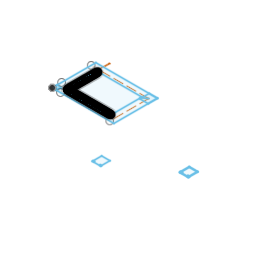
2023_01_21_LaserA4Measure (Autodesk Fusion 360 design; units mm, degrees)
Autodesk Fusion 360 part; units mm, degrees
sketch "Esquisse1" plane through (0, 0, 0) normal (0, 0, 1) x (1, 0, 0)
  line L0 (0, 0) -> (40, 0)
  line L1 (40, 0) -> (40, 45)
  line L2 (40, 45) -> (0, 45)
  line L3 (0, 45) -> (0, 0)
  line L4 (20, 43) -> (20, 40.2)
  line L5 (20, 43) -> (0, 43)
  line L6 (0, 43) -> (0, 45)
  line L7 (0, 45) -> (20, 45)
  line L8 (20, 45) -> (20, 43)
  line L9 (20, 43) -> (40, 43)
  line L10 (40, 43) -> (40, 45)
  line L11 (40, 45) -> (20, 45)
  line L12 (20, 45) -> (20, 43)
  line L13 (20, 43) -> (40, 43)
  line L14 (40, 43) -> (40, 40.2)
  line L15 (40, 40.2) -> (20, 40.2)
  line L16 (20, 40.2) -> (20, 43)
  line L17 (20, 43) -> (0, 43)
  line L18 (0, 43) -> (0, 40.2)
  line L19 (20, 40.2) -> (20, 43)
  line L20 (-0.3, 45.3) -> (-0.3, -0.3)
  line L21 (-0.3, -0.3) -> (40.3, -0.3)
  line L22 (40.3, -0.3) -> (40.3, 45.3)
  line L23 (40.3, 45.3) -> (20, 45.3)
  line L24 (-0.3, 45.3) -> (20, 45.3)
  line L25 (20, 41.6) -> (5.56, 41.6)
  line L26 (20, 41.6) -> (34.44, 41.6)
  line L27 (34.44, 40.2) -> (34.44, 43)
  line L28 (-4.5858, 40) -> (-4.5858, 43)
  line L29 (5.56, 40.2) -> (5.56, 43)
  line L30 (20, 40.2) -> (-0.0001, 40.2)
  dimension "d1" = 40
  dimension "d2" = 45
  dimension "d7" = 2.8
  dimension "d8" = 2
  dimension "d9" = -0.3
  dimension "d10" = 14.44
  dimension "d11" = 14.44
  dimension "d12" = 3
  constraint horizontal L0
  constraint vertical L1
  constraint horizontal L2
  constraint vertical L3
  constraint coincident L0.start L3.end
  constraint vertical L4
  constraint horizontal L5
  constraint vertical L6
  constraint horizontal L7
  constraint vertical L8
  constraint horizontal L9
  constraint vertical L10
  constraint horizontal L11
  constraint vertical L12
  constraint horizontal L13
  constraint vertical L14
  constraint horizontal L15
  constraint vertical L16
  constraint coincident L1 L14.end
  constraint horizontal L17
  constraint vertical L18
  constraint vertical L19
  constraint midpoint L4 L25.start
  constraint perpendicular L16 L25
  constraint perpendicular L19 L26
  constraint coincident L15 L27.start
  constraint perpendicular L15 L27
  constraint coincident L5 L28.end
  constraint perpendicular L5 L28
  constraint coincident L5 L29.end
  constraint perpendicular L5 L29
  constraint horizontal L30
  constraint coincident L30 L29.start
  constraint coincident L30 L18.end
  measures "d1" distance of L0.start L0.end
  measures "d2" distance of L0.start L2.end
  measures "d7" distance of L4.start L4.end
  measures "d8" distance of L4.start L7.end
  measures "d10" distance of L25.start L25.end
  measures "d11" distance of L25.start L26.end
  measures "d12" distance of L28.start L28.end
extrude "Extrusion1" add sketch "Esquisse1" along normal blind 2 contours L0 L1 L3 L15 L30 | L2 L3 L5 L6 L7 L8 L12 L17 | L4 L16 L19 L25 L29 L30 | L1 L2 L8 L9 L10 L11 L12 L13 | L4 L15 L16 L19 L26 L27 | L4 L5 L16 L17 L19 L25 L29 | L4 L9 L13 L16 L19 L26 L27 makes body 1
sketch "Esquisse2" plane through (0, 0, 2) normal (0, 0, 1) x (-1, 0, 0)
  line L0 (0, -40.2) -> (0, 0)
  line L1 (0, 0) -> (-40, 0)
  line L2 (-40, 0) -> (-40, -40.2)
  line L3 (-40, -40.2) -> (-34.44, -40.2)
  line L4 (-34.44, -40.2) -> (-34.44, -43)
  line L5 (-34.44, -43) -> (-40, -43)
  line L6 (-40, -43) -> (-40, -45)
  line L7 (-40, -45) -> (0, -45)
  line L8 (0, -45) -> (0, -43)
  line L9 (0, -43) -> (-5.56, -43)
  line L10 (-5.56, -43) -> (-5.56, -40.2)
  line L11 (-5.56, -40.2) -> (0, -40.2)
  line L12 (-34.74, -40.5) -> (-34.74, -42.7)
  line L13 (-34.74, -42.7) -> (-40.3, -42.7)
  line L14 (-40.3, -42.7) -> (-40.3, -45.3)
  line L15 (-40.3, -45.3) -> (0.3, -45.3)
  line L16 (0.3, -45.3) -> (0.3, -42.7)
  line L17 (0.3, -42.7) -> (-5.26, -42.7)
  line L18 (-5.26, -42.7) -> (-5.26, -40.5)
  line L19 (-5.26, -40.5) -> (0.3, -40.5)
  line L20 (0.3, -40.5) -> (0.3, 0.3)
  line L21 (0.3, 0.3) -> (-40.3, 0.3)
  line L22 (-40.3, 0.3) -> (-40.3, -40.5)
  line L23 (-40.3, -40.5) -> (-34.74, -40.5)
  line L24 (-44, -39) -> (-44, -44.2)
  line L25 (-44, -44.2) -> (-44, -49)
  line L26 (-44, -49) -> (4, -49)
  line L27 (4, -49) -> (4, -44.2)
  line L28 (4, -44.2) -> (4, -39)
  line L29 (4, -39) -> (4, 4)
  line L30 (4, 4) -> (-44, 4)
  line L31 (-44, 4) -> (-44, -39)
  dimension "d15" = 0.3
  dimension "d16" = 4
extrude "Extrusion2" add sketch "Esquisse2" against normal blind 2 separate body contours L24 L25 L26 L27 L28 L29 L30 L31 makes body 2
sketch "Esquisse3" plane through (0, 0, 0) normal (0, 0, 1) x (1, 0, 0)
  line L0 (0, 0) -> (410, 0)
  line L1 (410, 0) -> (410, 400)
  line L2 (410, 400) -> (0, 400)
  line L3 (0, 400) -> (0, 0)
  line L4 (10, 10) -> (400, 10)
  line L5 (400, 10) -> (400, 390)
  line L6 (400, 390) -> (10, 390)
  line L7 (10, 390) -> (10, 10)
  dimension "d19" = 410
  dimension "d20" = 400
  dimension "d21" = -10
  constraint horizontal L0
  constraint vertical L1
  constraint horizontal L2
  constraint vertical L3
  constraint coincident L0.start L3.end
  measures "d19" distance of L0.start L0.end
  measures "d20" distance of L0.start L2.end
move_body "Déplacer1" bodies 1 2 to x (1, 0, 0) y (0, 1, 0) z (0, 0, 1) at (20, 20, 0)
sketch "Esquisse4" plane through (0, 0, 2) normal (0, 0, 1) x (-1, 0, 0)
  line L0 (-20, -60.2) -> (-20, -20)
  line L1 (-20, -20) -> (-60, -20)
  line L2 (-60, -20) -> (-60, -60.2)
  line L3 (-60, -60.2) -> (-54.44, -60.2)
  line L4 (-54.44, -60.2) -> (-54.44, -63)
  line L5 (-54.44, -63) -> (-60, -63)
  line L6 (-60, -63) -> (-60, -65)
  line L7 (-60, -65) -> (-20, -65)
  line L8 (-20, -65) -> (-20, -63)
  line L9 (-20, -63) -> (-25.56, -63)
  line L10 (-25.56, -63) -> (-25.56, -60.2)
  line L11 (-25.56, -60.2) -> (-20, -60.2)
copy_body "Copier/Coller des corps1" bodies 2 1 makes body 3 makes body 4
move_body "Déplacer2" bodies 3 4 to x (1, 0, 0) y (0, 1, 0) z (0, 0, 1) at (300, 300, 0)
sketch "Esquisse5" plane through (0, 0, 0) normal (0, 0, 1) x (1, 0, 0)
  line L0 (-350, 0) -> (-53, 0)
  line L1 (-53, 0) -> (-53, 210)
  line L2 (-53, 210) -> (-350, 210)
  line L3 (-350, 210) -> (-350, 0)
  line L4 (-345, 5) -> (-58, 5)
  line L5 (-58, 5) -> (-58, 205)
  line L6 (-58, 205) -> (-345, 205)
  line L7 (-345, 205) -> (-345, 5)
  line L8 (-305.6385, 29.0688) -> (-95.6385, 29.0688)
  line L9 (-95.6385, 29.0688) -> (-95.6385, 177.5688)
  line L10 (-95.6385, 177.5688) -> (-305.6385, 177.5688)
  line L11 (-305.6385, 177.5688) -> (-305.6385, 29.0688)
  dimension "d28" = 297
  dimension "d29" = 210
  dimension "d30" = -5
  dimension "d31" = 210
  dimension "d32" = 148.5
  constraint horizontal L0
  constraint vertical L1
  constraint horizontal L2
  constraint vertical L3
  constraint horizontal L8
  constraint vertical L9
  constraint horizontal L10
  constraint vertical L11
  measures "d28" distance of L0.start L0.end
  measures "d29" distance of L0.start L2.end
  measures "d31" distance of L8.start L8.end
  measures "d32" distance of L8.start L10.end
copy_body "Copier/Coller des corps2" bodies 1 makes body 5
move_body "Déplacer3" bodies 5 to x (1, 0, 0) y (0, 1, 0) z (0, 0, 1) at (-370, -20, 0)
copy_body "Copier/Coller des corps3" bodies 5 makes body 6
move_body "Déplacer4" bodies 6 to x (1, 0, 0) y (0, 1, 0) z (0, 0, 1) at (257, 165, 0)
sketch "Esquisse7" plane through (0, 0, 2) normal (0, 0, 1) x (-1, 0, 0)
  line L0 (350, -40.2) -> (350, 0)
  line L1 (350, 0) -> (310, 0)
  line L2 (310, 0) -> (310, -40.2)
  line L3 (310, -40.2) -> (315.56, -40.2)
  line L4 (315.56, -40.2) -> (315.56, -43)
  line L5 (315.56, -43) -> (310, -43)
  line L6 (310, -43) -> (310, -45)
  line L7 (310, -45) -> (350, -45)
  line L8 (350, -45) -> (350, -43)
  line L9 (350, -43) -> (344.44, -43)
  line L10 (344.44, -43) -> (344.44, -40.2)
  line L11 (344.44, -40.2) -> (350, -40.2)
  line L12 (350, -43) -> (344.44, -43)
  line L13 (344.44, -43) -> (344.44, -40.2)
  line L14 (344.44, -40.2) -> (350, -40.2)
  line L15 (350, -40.2) -> (350, 0)
  line L16 (350, 0) -> (310, 0)
  line L17 (310, 0) -> (310, -40.2)
  line L18 (310, -40.2) -> (315.56, -40.2)
  line L19 (315.56, -40.2) -> (315.56, -43)
  line L20 (315.56, -43) -> (310, -43)
  line L21 (310, -43) -> (310, -45)
  line L22 (310, -45) -> (350, -45)
  line L23 (350, -45) -> (350, -43)
sketch "Esquisse8" plane through (0, 0, 2) normal (0, 0, 1) x (-1, 0, 0)
  line L0 (93, -205.2) -> (93, -165)
  line L1 (93, -165) -> (53, -165)
  line L2 (53, -165) -> (53, -205.2)
  line L3 (53, -205.2) -> (58.56, -205.2)
  line L4 (58.56, -205.2) -> (58.56, -208)
  line L5 (58.56, -208) -> (53, -208)
  line L6 (53, -208) -> (53, -210)
  line L7 (53, -210) -> (93, -210)
  line L8 (93, -210) -> (93, -208)
  line L9 (93, -208) -> (87.44, -208)
  line L10 (87.44, -208) -> (87.44, -205.2)
  line L11 (87.44, -205.2) -> (93, -205.2)
  line L12 (53, -205.2) -> (58.56, -205.2)
  line L13 (58.56, -205.2) -> (58.56, -208)
  line L14 (58.56, -208) -> (53, -208)
  line L15 (53, -208) -> (53, -210)
  line L16 (53, -210) -> (93, -210)
  line L17 (93, -210) -> (93, -208)
  line L18 (93, -208) -> (87.44, -208)
  line L19 (87.44, -208) -> (87.44, -205.2)
  line L20 (87.44, -205.2) -> (93, -205.2)
  line L21 (93, -205.2) -> (93, -165)
  line L22 (93, -165) -> (53, -165)
  line L23 (53, -165) -> (53, -205.2)
sketch "Esquisse6" plane through (0, 0, 0) normal (0, 0, 1) x (1, 0, 0)
  line L0 (-305.6385, 29.0688) -> (-305.6385, 20)
  line L1 (-295.6385, 29.0688) -> (-295.6385, 20)
  line L2 (-285.6385, 29.0688) -> (-285.6385, 20)
  line L3 (-275.6385, 29.0688) -> (-275.6385, 20)
  line L4 (-265.6385, 29.0688) -> (-265.6385, 20)
  line L5 (-255.6385, 29.0688) -> (-255.6385, 20)
  line L6 (-245.6385, 29.0688) -> (-245.6385, 20)
  line L7 (-235.6385, 29.0688) -> (-235.6385, 20)
  line L8 (-225.6385, 29.0688) -> (-225.6385, 20)
  line L9 (-215.6385, 29.0688) -> (-215.6385, 20)
  line L10 (-205.6385, 29.0688) -> (-205.6385, 20)
  line L11 (-195.6385, 29.0688) -> (-195.6385, 20)
  line L12 (-185.6385, 29.0688) -> (-185.6385, 20)
  line L13 (-175.6385, 29.0688) -> (-175.6385, 20)
  line L14 (-165.6385, 29.0688) -> (-165.6385, 20)
  line L15 (-155.6385, 29.0688) -> (-155.6385, 20)
  line L16 (-145.6385, 29.0688) -> (-145.6385, 20)
  line L17 (-135.6385, 29.0688) -> (-135.6385, 20)
  line L18 (-125.6385, 29.0688) -> (-125.6385, 20)
  line L19 (-115.6385, 29.0688) -> (-115.6385, 20)
  line L20 (-105.6385, 29.0688) -> (-105.6385, 20)
  line L21 (-95.6385, 29.0688) -> (-95.6385, 20)
  line L22 (-305.6385, 29.0688) -> (-305.6385, 27)
  line L23 (-304.6385, 29.0688) -> (-304.6385, 27)
  line L24 (-303.6385, 29.0688) -> (-303.6385, 27)
  line L25 (-302.6385, 29.0688) -> (-302.6385, 27)
  line L26 (-301.6385, 29.0688) -> (-301.6385, 27)
  line L27 (-300.6385, 29.0688) -> (-300.6385, 27)
  line L28 (-299.6385, 29.0688) -> (-299.6385, 27)
  line L29 (-298.6385, 29.0688) -> (-298.6385, 27)
  line L30 (-297.6385, 29.0688) -> (-297.6385, 27)
  line L31 (-296.6385, 29.0688) -> (-296.6385, 27)
  line L32 (-295.6385, 29.0688) -> (-295.6385, 27)
  line L33 (-294.6385, 29.0688) -> (-294.6385, 27)
  line L34 (-293.6385, 29.0688) -> (-293.6385, 27)
  line L35 (-292.6385, 29.0688) -> (-292.6385, 27)
  line L36 (-291.6385, 29.0688) -> (-291.6385, 27)
  line L37 (-290.6385, 29.0688) -> (-290.6385, 27)
  line L38 (-289.6385, 29.0688) -> (-289.6385, 27)
  line L39 (-288.6385, 29.0688) -> (-288.6385, 27)
  line L40 (-287.6385, 29.0688) -> (-287.6385, 27)
  line L41 (-286.6385, 29.0688) -> (-286.6385, 27)
  line L42 (-285.6385, 29.0688) -> (-285.6385, 27)
  line L43 (-284.6385, 29.0688) -> (-284.6385, 27)
  line L44 (-283.6385, 29.0688) -> (-283.6385, 27)
  line L45 (-282.6385, 29.0688) -> (-282.6385, 27)
  line L46 (-281.6385, 29.0688) -> (-281.6385, 27)
  line L47 (-280.6385, 29.0688) -> (-280.6385, 27)
  line L48 (-279.6385, 29.0688) -> (-279.6385, 27)
  line L49 (-278.6385, 29.0688) -> (-278.6385, 27)
  line L50 (-277.6385, 29.0688) -> (-277.6385, 27)
  line L51 (-276.6385, 29.0688) -> (-276.6385, 27)
  line L52 (-275.6385, 29.0688) -> (-275.6385, 27)
  line L53 (-274.6385, 29.0688) -> (-274.6385, 27)
  line L54 (-273.6385, 29.0688) -> (-273.6385, 27)
  line L55 (-272.6385, 29.0688) -> (-272.6385, 27)
  line L56 (-271.6385, 29.0688) -> (-271.6385, 27)
  line L57 (-270.6385, 29.0688) -> (-270.6385, 27)
  line L58 (-269.6385, 29.0688) -> (-269.6385, 27)
  line L59 (-268.6385, 29.0688) -> (-268.6385, 27)
  line L60 (-267.6385, 29.0688) -> (-267.6385, 27)
  line L61 (-266.6385, 29.0688) -> (-266.6385, 27)
  line L62 (-265.6385, 29.0688) -> (-265.6385, 27)
  line L63 (-264.6385, 29.0688) -> (-264.6385, 27)
  line L64 (-263.6385, 29.0688) -> (-263.6385, 27)
  line L65 (-262.6385, 29.0688) -> (-262.6385, 27)
  line L66 (-261.6385, 29.0688) -> (-261.6385, 27)
  line L67 (-260.6385, 29.0688) -> (-260.6385, 27)
  line L68 (-259.6385, 29.0688) -> (-259.6385, 27)
  line L69 (-258.6385, 29.0688) -> (-258.6385, 27)
  line L70 (-257.6385, 29.0688) -> (-257.6385, 27)
  line L71 (-256.6385, 29.0688) -> (-256.6385, 27)
  line L72 (-255.6385, 29.0688) -> (-255.6385, 27)
  line L73 (-254.6385, 29.0688) -> (-254.6385, 27)
  line L74 (-253.6385, 29.0688) -> (-253.6385, 27)
  line L75 (-252.6385, 29.0688) -> (-252.6385, 27)
  line L76 (-251.6385, 29.0688) -> (-251.6385, 27)
  line L77 (-250.6385, 29.0688) -> (-250.6385, 27)
  line L78 (-249.6385, 29.0688) -> (-249.6385, 27)
  line L79 (-248.6385, 29.0688) -> (-248.6385, 27)
  line L80 (-247.6385, 29.0688) -> (-247.6385, 27)
  line L81 (-246.6385, 29.0688) -> (-246.6385, 27)
  line L82 (-245.6385, 29.0688) -> (-245.6385, 27)
  line L83 (-244.6385, 29.0688) -> (-244.6385, 27)
  line L84 (-243.6385, 29.0688) -> (-243.6385, 27)
  line L85 (-242.6385, 29.0688) -> (-242.6385, 27)
  line L86 (-241.6385, 29.0688) -> (-241.6385, 27)
  line L87 (-240.6385, 29.0688) -> (-240.6385, 27)
  line L88 (-239.6385, 29.0688) -> (-239.6385, 27)
  line L89 (-238.6385, 29.0688) -> (-238.6385, 27)
  line L90 (-237.6385, 29.0688) -> (-237.6385, 27)
  line L91 (-236.6385, 29.0688) -> (-236.6385, 27)
  line L92 (-235.6385, 29.0688) -> (-235.6385, 27)
  line L93 (-234.6385, 29.0688) -> (-234.6385, 27)
  line L94 (-233.6385, 29.0688) -> (-233.6385, 27)
  line L95 (-232.6385, 29.0688) -> (-232.6385, 27)
  line L96 (-231.6385, 29.0688) -> (-231.6385, 27)
  line L97 (-230.6385, 29.0688) -> (-230.6385, 27)
  line L98 (-229.6385, 29.0688) -> (-229.6385, 27)
  line L99 (-228.6385, 29.0688) -> (-228.6385, 27)
  line L100 (-227.6385, 29.0688) -> (-227.6385, 27)
  line L101 (-226.6385, 29.0688) -> (-226.6385, 27)
  line L102 (-225.6385, 29.0688) -> (-225.6385, 27)
  line L103 (-224.6385, 29.0688) -> (-224.6385, 27)
  line L104 (-223.6385, 29.0688) -> (-223.6385, 27)
  line L105 (-222.6385, 29.0688) -> (-222.6385, 27)
  line L106 (-221.6385, 29.0688) -> (-221.6385, 27)
  line L107 (-220.6385, 29.0688) -> (-220.6385, 27)
  line L108 (-219.6385, 29.0688) -> (-219.6385, 27)
  line L109 (-218.6385, 29.0688) -> (-218.6385, 27)
  line L110 (-217.6385, 29.0688) -> (-217.6385, 27)
  line L111 (-216.6385, 29.0688) -> (-216.6385, 27)
  line L112 (-215.6385, 29.0688) -> (-215.6385, 27)
  line L113 (-214.6385, 29.0688) -> (-214.6385, 27)
  line L114 (-213.6385, 29.0688) -> (-213.6385, 27)
  line L115 (-212.6385, 29.0688) -> (-212.6385, 27)
  line L116 (-211.6385, 29.0688) -> (-211.6385, 27)
  line L117 (-210.6385, 29.0688) -> (-210.6385, 27)
  line L118 (-209.6385, 29.0688) -> (-209.6385, 27)
  line L119 (-208.6385, 29.0688) -> (-208.6385, 27)
  line L120 (-207.6385, 29.0688) -> (-207.6385, 27)
  line L121 (-206.6385, 29.0688) -> (-206.6385, 27)
  line L122 (-205.6385, 29.0688) -> (-205.6385, 27)
  line L123 (-204.6385, 29.0688) -> (-204.6385, 27)
  line L124 (-203.6385, 29.0688) -> (-203.6385, 27)
  line L125 (-202.6385, 29.0688) -> (-202.6385, 27)
  line L126 (-201.6385, 29.0688) -> (-201.6385, 27)
  line L127 (-200.6385, 29.0688) -> (-200.6385, 27)
  line L128 (-199.6385, 29.0688) -> (-199.6385, 27)
  line L129 (-198.6385, 29.0688) -> (-198.6385, 27)
  line L130 (-197.6385, 29.0688) -> (-197.6385, 27)
  line L131 (-196.6385, 29.0688) -> (-196.6385, 27)
  line L132 (-195.6385, 29.0688) -> (-195.6385, 27)
  line L133 (-194.6385, 29.0688) -> (-194.6385, 27)
  line L134 (-193.6385, 29.0688) -> (-193.6385, 27)
  line L135 (-192.6385, 29.0688) -> (-192.6385, 27)
  line L136 (-191.6385, 29.0688) -> (-191.6385, 27)
  line L137 (-190.6385, 29.0688) -> (-190.6385, 27)
  line L138 (-189.6385, 29.0688) -> (-189.6385, 27)
  line L139 (-188.6385, 29.0688) -> (-188.6385, 27)
  line L140 (-187.6385, 29.0688) -> (-187.6385, 27)
  line L141 (-186.6385, 29.0688) -> (-186.6385, 27)
  line L142 (-185.6385, 29.0688) -> (-185.6385, 27)
  line L143 (-184.6385, 29.0688) -> (-184.6385, 27)
  line L144 (-183.6385, 29.0688) -> (-183.6385, 27)
  line L145 (-182.6385, 29.0688) -> (-182.6385, 27)
  line L146 (-181.6385, 29.0688) -> (-181.6385, 27)
  line L147 (-180.6385, 29.0688) -> (-180.6385, 27)
  line L148 (-179.6385, 29.0688) -> (-179.6385, 27)
  line L149 (-178.6385, 29.0688) -> (-178.6385, 27)
  line L150 (-177.6385, 29.0688) -> (-177.6385, 27)
  line L151 (-176.6385, 29.0688) -> (-176.6385, 27)
  line L152 (-175.6385, 29.0688) -> (-175.6385, 27)
  line L153 (-174.6385, 29.0688) -> (-174.6385, 27)
  line L154 (-173.6385, 29.0688) -> (-173.6385, 27)
  line L155 (-172.6385, 29.0688) -> (-172.6385, 27)
  line L156 (-171.6385, 29.0688) -> (-171.6385, 27)
  line L157 (-170.6385, 29.0688) -> (-170.6385, 27)
  line L158 (-169.6385, 29.0688) -> (-169.6385, 27)
  line L159 (-168.6385, 29.0688) -> (-168.6385, 27)
  line L160 (-167.6385, 29.0688) -> (-167.6385, 27)
  line L161 (-166.6385, 29.0688) -> (-166.6385, 27)
  line L162 (-165.6385, 29.0688) -> (-165.6385, 27)
  line L163 (-164.6385, 29.0688) -> (-164.6385, 27)
  line L164 (-163.6385, 29.0688) -> (-163.6385, 27)
  line L165 (-162.6385, 29.0688) -> (-162.6385, 27)
  line L166 (-161.6385, 29.0688) -> (-161.6385, 27)
  line L167 (-160.6385, 29.0688) -> (-160.6385, 27)
  line L168 (-159.6385, 29.0688) -> (-159.6385, 27)
  line L169 (-158.6385, 29.0688) -> (-158.6385, 27)
  line L170 (-157.6385, 29.0688) -> (-157.6385, 27)
  line L171 (-156.6385, 29.0688) -> (-156.6385, 27)
  line L172 (-155.6385, 29.0688) -> (-155.6385, 27)
  line L173 (-154.6385, 29.0688) -> (-154.6385, 27)
  line L174 (-153.6385, 29.0688) -> (-153.6385, 27)
  line L175 (-152.6385, 29.0688) -> (-152.6385, 27)
  line L176 (-151.6385, 29.0688) -> (-151.6385, 27)
  line L177 (-150.6385, 29.0688) -> (-150.6385, 27)
  line L178 (-149.6385, 29.0688) -> (-149.6385, 27)
  line L179 (-148.6385, 29.0688) -> (-148.6385, 27)
  line L180 (-147.6385, 29.0688) -> (-147.6385, 27)
  line L181 (-146.6385, 29.0688) -> (-146.6385, 27)
  line L182 (-145.6385, 29.0688) -> (-145.6385, 27)
  line L183 (-144.6385, 29.0688) -> (-144.6385, 27)
  line L184 (-143.6385, 29.0688) -> (-143.6385, 27)
  line L185 (-142.6385, 29.0688) -> (-142.6385, 27)
  line L186 (-141.6385, 29.0688) -> (-141.6385, 27)
  line L187 (-140.6385, 29.0688) -> (-140.6385, 27)
  line L188 (-139.6385, 29.0688) -> (-139.6385, 27)
  line L189 (-138.6385, 29.0688) -> (-138.6385, 27)
  line L190 (-137.6385, 29.0688) -> (-137.6385, 27)
  line L191 (-136.6385, 29.0688) -> (-136.6385, 27)
  line L192 (-135.6385, 29.0688) -> (-135.6385, 27)
  line L193 (-134.6385, 29.0688) -> (-134.6385, 27)
  line L194 (-133.6385, 29.0688) -> (-133.6385, 27)
  line L195 (-132.6385, 29.0688) -> (-132.6385, 27)
  line L196 (-131.6385, 29.0688) -> (-131.6385, 27)
  line L197 (-130.6385, 29.0688) -> (-130.6385, 27)
  line L198 (-129.6385, 29.0688) -> (-129.6385, 27)
  line L199 (-128.6385, 29.0688) -> (-128.6385, 27)
  line L200 (-127.6385, 29.0688) -> (-127.6385, 27)
  line L201 (-126.6385, 29.0688) -> (-126.6385, 27)
  line L202 (-125.6385, 29.0688) -> (-125.6385, 27)
  line L203 (-124.6385, 29.0688) -> (-124.6385, 27)
  line L204 (-123.6385, 29.0688) -> (-123.6385, 27)
  line L205 (-122.6385, 29.0688) -> (-122.6385, 27)
  line L206 (-121.6385, 29.0688) -> (-121.6385, 27)
  line L207 (-120.6385, 29.0688) -> (-120.6385, 27)
  line L208 (-119.6385, 29.0688) -> (-119.6385, 27)
  line L209 (-118.6385, 29.0688) -> (-118.6385, 27)
  line L210 (-117.6385, 29.0688) -> (-117.6385, 27)
  line L211 (-116.6385, 29.0688) -> (-116.6385, 27)
  line L212 (-115.6385, 29.0688) -> (-115.6385, 27)
  line L213 (-114.6385, 29.0688) -> (-114.6385, 27)
  line L214 (-113.6385, 29.0688) -> (-113.6385, 27)
  line L215 (-112.6385, 29.0688) -> (-112.6385, 27)
  line L216 (-111.6385, 29.0688) -> (-111.6385, 27)
  line L217 (-110.6385, 29.0688) -> (-110.6385, 27)
  line L218 (-109.6385, 29.0688) -> (-109.6385, 27)
  line L219 (-108.6385, 29.0688) -> (-108.6385, 27)
  line L220 (-107.6385, 29.0688) -> (-107.6385, 27)
  line L221 (-106.6385, 29.0688) -> (-106.6385, 27)
  line L222 (-105.6385, 29.0688) -> (-105.6385, 27)
  line L223 (-104.6385, 29.0688) -> (-104.6385, 27)
  line L224 (-103.6385, 29.0688) -> (-103.6385, 27)
  line L225 (-102.6385, 29.0688) -> (-102.6385, 27)
  line L226 (-101.6385, 29.0688) -> (-101.6385, 27)
  line L227 (-100.6385, 29.0688) -> (-100.6385, 27)
  line L228 (-99.6385, 29.0688) -> (-99.6385, 27)
  line L229 (-98.6385, 29.0688) -> (-98.6385, 27)
  line L230 (-97.6385, 29.0688) -> (-97.6385, 27)
  line L231 (-96.6385, 29.0688) -> (-96.6385, 27)
  line L232 (-305.6385, 29.0688) -> (-310, 29.0688)
  line L233 (-305.6385, 29.0688) -> (-307.7074, 29.0688)
  line L234 (-305.6385, 30.0688) -> (-307.7074, 30.0688)
  line L235 (-305.6385, 31.0688) -> (-307.7074, 31.0688)
  line L236 (-305.6385, 32.0688) -> (-307.7074, 32.0688)
  line L237 (-305.6385, 33.0688) -> (-307.7074, 33.0688)
  line L238 (-305.6385, 34.0688) -> (-307.7074, 34.0688)
  line L239 (-305.6385, 35.0688) -> (-307.7074, 35.0688)
  line L240 (-305.6385, 36.0688) -> (-307.7074, 36.0688)
  line L241 (-305.6385, 37.0688) -> (-307.7074, 37.0688)
  line L242 (-305.6385, 38.0688) -> (-307.7074, 38.0688)
  line L243 (-305.6385, 39.0688) -> (-307.7074, 39.0688)
  line L244 (-305.6385, 40.0688) -> (-307.7074, 40.0688)
  line L245 (-305.6385, 41.0688) -> (-307.7074, 41.0688)
  line L246 (-305.6385, 42.0688) -> (-307.7074, 42.0688)
  line L247 (-305.6385, 43.0688) -> (-307.7074, 43.0688)
  line L248 (-305.6385, 44.0688) -> (-307.7074, 44.0688)
  line L249 (-305.6385, 45.0688) -> (-307.7074, 45.0688)
  line L250 (-305.6385, 46.0688) -> (-307.7074, 46.0688)
  line L251 (-305.6385, 47.0688) -> (-307.7074, 47.0688)
  line L252 (-305.6385, 48.0688) -> (-307.7074, 48.0688)
  line L253 (-305.6385, 49.0688) -> (-307.7074, 49.0688)
  line L254 (-305.6385, 50.0688) -> (-307.7074, 50.0688)
  line L255 (-305.6385, 51.0688) -> (-307.7074, 51.0688)
  line L256 (-305.6385, 52.0688) -> (-307.7074, 52.0688)
  line L257 (-305.6385, 53.0688) -> (-307.7074, 53.0688)
  line L258 (-305.6385, 54.0688) -> (-307.7074, 54.0688)
  line L259 (-305.6385, 55.0688) -> (-307.7074, 55.0688)
  line L260 (-305.6385, 56.0688) -> (-307.7074, 56.0688)
  line L261 (-305.6385, 57.0688) -> (-307.7074, 57.0688)
  line L262 (-305.6385, 58.0688) -> (-307.7074, 58.0688)
  line L263 (-305.6385, 59.0688) -> (-307.7074, 59.0688)
  line L264 (-305.6385, 60.0688) -> (-307.7074, 60.0688)
  line L265 (-305.6385, 61.0688) -> (-307.7074, 61.0688)
  line L266 (-305.6385, 62.0688) -> (-307.7074, 62.0688)
  line L267 (-305.6385, 63.0688) -> (-307.7074, 63.0688)
  line L268 (-305.6385, 64.0688) -> (-307.7074, 64.0688)
  line L269 (-305.6385, 65.0688) -> (-307.7074, 65.0688)
  line L270 (-305.6385, 66.0688) -> (-307.7074, 66.0688)
  line L271 (-305.6385, 67.0688) -> (-307.7074, 67.0688)
  line L272 (-305.6385, 68.0688) -> (-307.7074, 68.0688)
  line L273 (-305.6385, 69.0688) -> (-307.7074, 69.0688)
  line L274 (-305.6385, 70.0688) -> (-307.7074, 70.0688)
  line L275 (-305.6385, 71.0688) -> (-307.7074, 71.0688)
  line L276 (-305.6385, 72.0688) -> (-307.7074, 72.0688)
  line L277 (-305.6385, 73.0688) -> (-307.7074, 73.0688)
  line L278 (-305.6385, 74.0688) -> (-307.7074, 74.0688)
  line L279 (-305.6385, 75.0688) -> (-307.7074, 75.0688)
  line L280 (-305.6385, 76.0688) -> (-307.7074, 76.0688)
  line L281 (-305.6385, 77.0688) -> (-307.7074, 77.0688)
  line L282 (-305.6385, 78.0688) -> (-307.7074, 78.0688)
  line L283 (-305.6385, 79.0688) -> (-307.7074, 79.0688)
  line L284 (-305.6385, 80.0688) -> (-307.7074, 80.0688)
  line L285 (-305.6385, 81.0688) -> (-307.7074, 81.0688)
  line L286 (-305.6385, 82.0688) -> (-307.7074, 82.0688)
  line L287 (-305.6385, 83.0688) -> (-307.7074, 83.0688)
  line L288 (-305.6385, 84.0688) -> (-307.7074, 84.0688)
  line L289 (-305.6385, 85.0688) -> (-307.7074, 85.0688)
  line L290 (-305.6385, 86.0688) -> (-307.7074, 86.0688)
  line L291 (-305.6385, 87.0688) -> (-307.7074, 87.0688)
  line L292 (-305.6385, 88.0688) -> (-307.7074, 88.0688)
  line L293 (-305.6385, 89.0688) -> (-307.7074, 89.0688)
  line L294 (-305.6385, 90.0688) -> (-307.7074, 90.0688)
  line L295 (-305.6385, 91.0688) -> (-307.7074, 91.0688)
  line L296 (-305.6385, 92.0688) -> (-307.7074, 92.0688)
  line L297 (-305.6385, 93.0688) -> (-307.7074, 93.0688)
  line L298 (-305.6385, 94.0688) -> (-307.7074, 94.0688)
  line L299 (-305.6385, 95.0688) -> (-307.7074, 95.0688)
  line L300 (-305.6385, 96.0688) -> (-307.7074, 96.0688)
  line L301 (-305.6385, 97.0688) -> (-307.7074, 97.0688)
  line L302 (-305.6385, 98.0688) -> (-307.7074, 98.0688)
  line L303 (-305.6385, 99.0688) -> (-307.7074, 99.0688)
  line L304 (-305.6385, 100.0688) -> (-307.7074, 100.0688)
  line L305 (-305.6385, 101.0688) -> (-307.7074, 101.0688)
  line L306 (-305.6385, 102.0688) -> (-307.7074, 102.0688)
  line L307 (-305.6385, 103.0688) -> (-307.7074, 103.0688)
  line L308 (-305.6385, 104.0688) -> (-307.7074, 104.0688)
  line L309 (-305.6385, 105.0688) -> (-307.7074, 105.0688)
  line L310 (-305.6385, 106.0688) -> (-307.7074, 106.0688)
  line L311 (-305.6385, 107.0688) -> (-307.7074, 107.0688)
  line L312 (-305.6385, 108.0688) -> (-307.7074, 108.0688)
  line L313 (-305.6385, 109.0688) -> (-307.7074, 109.0688)
  line L314 (-305.6385, 110.0688) -> (-307.7074, 110.0688)
  line L315 (-305.6385, 111.0688) -> (-307.7074, 111.0688)
  line L316 (-305.6385, 112.0688) -> (-307.7074, 112.0688)
  line L317 (-305.6385, 113.0688) -> (-307.7074, 113.0688)
  line L318 (-305.6385, 114.0688) -> (-307.7074, 114.0688)
  line L319 (-305.6385, 115.0688) -> (-307.7074, 115.0688)
  line L320 (-305.6385, 116.0688) -> (-307.7074, 116.0688)
  line L321 (-305.6385, 117.0688) -> (-307.7074, 117.0688)
  line L322 (-305.6385, 118.0688) -> (-307.7074, 118.0688)
  line L323 (-305.6385, 119.0688) -> (-307.7074, 119.0688)
  line L324 (-305.6385, 120.0688) -> (-307.7074, 120.0688)
  line L325 (-305.6385, 121.0688) -> (-307.7074, 121.0688)
  line L326 (-305.6385, 122.0688) -> (-307.7074, 122.0688)
  line L327 (-305.6385, 123.0688) -> (-307.7074, 123.0688)
  line L328 (-305.6385, 124.0688) -> (-307.7074, 124.0688)
  line L329 (-305.6385, 125.0688) -> (-307.7074, 125.0688)
  line L330 (-305.6385, 126.0688) -> (-307.7074, 126.0688)
  line L331 (-305.6385, 127.0688) -> (-307.7074, 127.0688)
  line L332 (-305.6385, 128.0688) -> (-307.7074, 128.0688)
  line L333 (-305.6385, 129.0688) -> (-307.7074, 129.0688)
  line L334 (-305.6385, 130.0688) -> (-307.7074, 130.0688)
  line L335 (-305.6385, 131.0688) -> (-307.7074, 131.0688)
  line L336 (-305.6385, 132.0688) -> (-307.7074, 132.0688)
  line L337 (-305.6385, 133.0688) -> (-307.7074, 133.0688)
  line L338 (-305.6385, 134.0688) -> (-307.7074, 134.0688)
  line L339 (-305.6385, 135.0688) -> (-307.7074, 135.0688)
  line L340 (-305.6385, 136.0688) -> (-307.7074, 136.0688)
  line L341 (-305.6385, 137.0688) -> (-307.7074, 137.0688)
  line L342 (-305.6385, 138.0688) -> (-307.7074, 138.0688)
  line L343 (-305.6385, 139.0688) -> (-307.7074, 139.0688)
  line L344 (-305.6385, 140.0688) -> (-307.7074, 140.0688)
  line L345 (-305.6385, 141.0688) -> (-307.7074, 141.0688)
  line L346 (-305.6385, 142.0688) -> (-307.7074, 142.0688)
  line L347 (-305.6385, 143.0688) -> (-307.7074, 143.0688)
  line L348 (-305.6385, 144.0688) -> (-307.7074, 144.0688)
  line L349 (-305.6385, 145.0688) -> (-307.7074, 145.0688)
  line L350 (-305.6385, 146.0688) -> (-307.7074, 146.0688)
  line L351 (-305.6385, 147.0688) -> (-307.7074, 147.0688)
  line L352 (-305.6385, 148.0688) -> (-307.7074, 148.0688)
  line L353 (-305.6385, 149.0688) -> (-307.7074, 149.0688)
  line L354 (-305.6385, 150.0688) -> (-307.7074, 150.0688)
  line L355 (-305.6385, 151.0688) -> (-307.7074, 151.0688)
  line L356 (-305.6385, 152.0688) -> (-307.7074, 152.0688)
  line L357 (-305.6385, 153.0688) -> (-307.7074, 153.0688)
  line L358 (-305.6385, 154.0688) -> (-307.7074, 154.0688)
  line L359 (-305.6385, 155.0688) -> (-307.7074, 155.0688)
  line L360 (-305.6385, 156.0688) -> (-307.7074, 156.0688)
  line L361 (-305.6385, 157.0688) -> (-307.7074, 157.0688)
  line L362 (-305.6385, 158.0688) -> (-307.7074, 158.0688)
  line L363 (-305.6385, 159.0688) -> (-307.7074, 159.0688)
  line L364 (-305.6385, 160.0688) -> (-307.7074, 160.0688)
  line L365 (-305.6385, 161.0688) -> (-307.7074, 161.0688)
  line L366 (-305.6385, 162.0688) -> (-307.7074, 162.0688)
  line L367 (-305.6385, 163.0688) -> (-307.7074, 163.0688)
  line L368 (-305.6385, 164.0688) -> (-307.7074, 164.0688)
  line L369 (-305.6385, 165.0688) -> (-307.7074, 165.0688)
  line L370 (-305.6385, 166.0688) -> (-307.7074, 166.0688)
  line L371 (-305.6385, 167.0688) -> (-307.7074, 167.0688)
  line L372 (-305.6385, 168.0688) -> (-307.7074, 168.0688)
  line L373 (-305.6385, 169.0688) -> (-307.7074, 169.0688)
  line L374 (-305.6385, 170.0688) -> (-307.7074, 170.0688)
  line L375 (-305.6385, 171.0688) -> (-307.7074, 171.0688)
  line L376 (-305.6385, 172.0688) -> (-307.7074, 172.0688)
  line L377 (-305.6385, 173.0688) -> (-307.7074, 173.0688)
  line L378 (-305.6385, 174.0688) -> (-307.7074, 174.0688)
  line L379 (-305.6385, 175.0688) -> (-307.7074, 175.0688)
  line L380 (-305.6385, 176.0688) -> (-307.7074, 176.0688)
  line L381 (-295.6385, 29.0688) -> (-300, 29.0688)
  line L382 (-285.6385, 29.0688) -> (-290, 29.0688)
  line L383 (-275.6385, 29.0688) -> (-280, 29.0688)
  line L384 (-265.6385, 29.0688) -> (-270, 29.0688)
  line L385 (-255.6385, 29.0688) -> (-260, 29.0688)
  line L386 (-245.6385, 29.0688) -> (-250, 29.0688)
  line L387 (-235.6385, 29.0688) -> (-240, 29.0688)
  line L388 (-225.6385, 29.0688) -> (-230, 29.0688)
  line L389 (-215.6385, 29.0688) -> (-220, 29.0688)
  line L390 (-205.6385, 29.0688) -> (-210, 29.0688)
  line L391 (-195.6385, 29.0688) -> (-200, 29.0688)
  line L392 (-185.6385, 29.0688) -> (-190, 29.0688)
  line L393 (-175.6385, 29.0688) -> (-180, 29.0688)
  line L394 (-165.6385, 29.0688) -> (-170, 29.0688)
  line L395 (-155.6385, 29.0688) -> (-160, 29.0688)
  line L396 (-305.6385, 39.0688) -> (-310, 39.0688)
  line L397 (-305.6385, 49.0688) -> (-310, 49.0688)
  line L398 (-305.6385, 59.0688) -> (-310, 59.0688)
  line L399 (-305.6385, 69.0688) -> (-310, 69.0688)
  line L400 (-305.6385, 79.0688) -> (-310, 79.0688)
  line L401 (-305.6385, 89.0688) -> (-310, 89.0688)
  line L402 (-305.6385, 99.0688) -> (-310, 99.0688)
  line L403 (-305.6385, 109.0688) -> (-310, 109.0688)
  line L404 (-305.6385, 119.0688) -> (-310, 119.0688)
  line L405 (-305.6385, 129.0688) -> (-310, 129.0688)
  line L406 (-305.6385, 139.0688) -> (-310, 139.0688)
  line L407 (-305.6385, 149.0688) -> (-310, 149.0688)
  line L408 (-305.6385, 159.0688) -> (-310, 159.0688)
  line L409 (-305.6385, 169.0688) -> (-310, 169.0688)
  line L410 (-305.6385, 15) -> (-95, 15) construction
  line L411 (-95, 15) -> (-95, 18.6119) construction
  line L412 (-95, 18.6119) -> (-305.6385, 18.6119) construction
  line L413 (-305.6385, 18.6119) -> (-305.6385, 15) construction
  line L414 (-311.7188, 29.1895) -> (-311.7188, 239.828) construction
  line L415 (-311.7188, 239.828) -> (-315.3307, 239.828) construction
  line L416 (-315.3307, 239.828) -> (-315.3307, 29.1895) construction
  line L417 (-315.3307, 29.1895) -> (-311.7188, 29.1895) construction
  line L418 (310, -40.2) -> (315.56, -40.2)
  line L419 (315.56, -40.2) -> (315.56, -43)
  line L420 (315.56, -43) -> (310, -43)
  line L421 (310, -43) -> (310, -45)
  line L422 (310, -45) -> (350, -45)
  line L423 (350, -45) -> (350, -43)
  line L424 (350, -43) -> (344.44, -43)
  line L425 (344.44, -43) -> (344.44, -40.2)
  line L426 (344.44, -40.2) -> (350, -40.2)
  line L427 (350, -40.2) -> (350, 0)
  line L428 (350, 0) -> (310, 0)
  line L429 (310, 0) -> (310, -40.2)
  line L430 (53, -205.2) -> (58.56, -205.2)
  line L431 (58.56, -205.2) -> (58.56, -208)
  line L432 (58.56, -208) -> (53, -208)
  line L433 (53, -208) -> (53, -210)
  line L434 (53, -210) -> (93, -210)
  line L435 (93, -210) -> (93, -208)
  line L436 (93, -208) -> (87.44, -208)
  line L437 (87.44, -208) -> (87.44, -205.2)
  line L438 (87.44, -205.2) -> (93, -205.2)
  line L439 (93, -205.2) -> (93, -165)
  line L440 (93, -165) -> (53, -165)
  line L441 (53, -165) -> (53, -205.2)
  line L442 (350, -43) -> (344.44, -43)
  line L443 (344.44, -43) -> (344.44, -40.2)
  line L444 (344.44, -40.2) -> (350, -40.2)
  line L445 (350, -40.2) -> (350, 0)
  line L446 (350, 0) -> (310, 0)
  line L447 (310, 0) -> (310, -40.2)
  line L448 (310, -40.2) -> (315.56, -40.2)
  line L449 (315.56, -40.2) -> (315.56, -43)
  line L450 (315.56, -43) -> (310, -43)
  line L451 (310, -43) -> (310, -45)
  line L452 (310, -45) -> (350, -45)
  line L453 (350, -45) -> (350, -43)
  line L454 (350, -43) -> (344.44, -43)
  line L455 (344.44, -43) -> (344.44, -40.2)
  line L456 (344.44, -40.2) -> (350, -40.2)
  line L457 (350, -40.2) -> (350, 0)
  line L458 (350, 0) -> (310, 0)
  line L459 (310, 0) -> (310, -40.2)
  line L460 (310, -40.2) -> (315.56, -40.2)
  line L461 (315.56, -40.2) -> (315.56, -43)
  line L462 (315.56, -43) -> (310, -43)
  line L463 (310, -43) -> (310, -45)
  line L464 (310, -45) -> (350, -45)
  line L465 (350, -45) -> (350, -43)
  line L466 (-310, 45.2638) -> (-310, 27.0773)
  line L467 (-310, 0) -> (-350, 0)
  line L468 (-53, 210) -> (-53, 165)
  line L469 (-53, 165) -> (-93.0303, 165)
  line L470 (-93.0303, 165) -> (-93.0303, 210)
  line L471 (-350, 0) -> (-350, 45.2638)
  line L472 (-93.0303, 210) -> (-53, 210)
  line L473 (-350, 22.6319) -> (-330, 22.6319)
  line L474 (-330, 22.6319) -> (-330, 0)
  line L475 (-73.0152, 187.5) -> (-97.9056, 170.6509)
  line L476 (-350, 0) -> (-321.971, 18.9738)
  line L477 (-326.7751, 5.0222) -> (-311.8896, 5.0418) construction
  line L478 (-311.8896, 5.0418) -> (-311.8995, 12.5287) construction
  line L479 (-311.8995, 12.5287) -> (-326.7849, 12.5091) construction
  line L480 (-326.7849, 12.5091) -> (-326.7751, 5.0222) construction
  line L481 (-73.0152, 187.5) -> (-73.0152, 0) construction
  line L482 (-73.0152, 187.5) -> (-350, 187.5) construction
  line L483 (-350, 0) -> (-330, 13.5386) construction
  line L484 (-310, 27.0773) -> (-307.058, 29.0688) construction
  line L485 (-93.0303, 173.9511) -> (-73.0152, 187.5) construction
  point P0 (-305.6385, 29.0688)
  point P1 (-350, 0)
  dimension "d41" = 10
  dimension "d42" = 0
  dimension "d45" = 1
  dimension "d46" = 0
  dimension "d49" = 0
  dimension "d50" = 1
  dimension "d53" = 10
  dimension "d54" = 10
  dimension "d55" = 3
  dimension "d56" = 3
  dimension "d62" = 2.5
  dimension "d63" = 187.5
  dimension "d64" = 276.9848
  constraint coincident P0 L0.start
  constraint coincident L0 L22.end
  constraint perpendicular L22 L232
  constraint coincident L232 L233.end
  constraint equal L23 L233
  constraint perpendicular L466 L467
  constraint perpendicular L467 L468
  constraint perpendicular L468 L469
  constraint perpendicular L468 L472
  constraint perpendicular L473 L474
  constraint coincident P1 L467.end
  constraint coincident L467 L474.end
  constraint coincident L471 L473.start
  constraint coincident L475.end L483
  constraint coincident L476.end L483
  constraint vertical L481
  constraint perpendicular L481 L482
  constraint coincident L474 L483.end
  constraint collinear L483 L484
  constraint coincident L232 L484.end
  constraint coincident L470 L485.start
  constraint collinear L484 L485
  measures "d63" distance of L475.start L481.end
  measures "d64" distance of L475.start L482.end
sketch "Esquisse9" plane through (0, 0, 0) normal (0, 0, 1) x (1, 0, 0)
  line L0 (-305.6385, 177.5688) -> (-305.6385, 29.0688)
  line L1 (-305.6385, 29.0688) -> (-95.6385, 29.0688)
  line L2 (-95.6385, 29.0688) -> (-95.6385, 177.5688)
  line L3 (-95.6385, 177.5688) -> (-305.6385, 177.5688)
  line L4 (-350, 210) -> (-350, 0)
  line L5 (-350, 0) -> (-53, 0)
  line L6 (-53, 0) -> (-53, 210)
  line L7 (-53, 210) -> (-350, 210)
  dimension "d58" = 210
  dimension "d59" = 148.5
  dimension "d60" = 297
  dimension "d61" = 210
  constraint horizontal L1
  constraint vertical L2
  constraint horizontal L3
  constraint vertical L0
  constraint horizontal L5
  constraint vertical L6
  constraint horizontal L7
  constraint vertical L4
  measures "d58" distance of L0.end L1.end
  measures "d59" distance of L0.start L0.end
  measures "d60" distance of L5.end L4.end
  measures "d61" distance of L4.end L4.start
sketch "Esquisse10" plane through (0, 0, 0) normal (0, 0, 1) x (1, 0, 0)
equation "d10 = ( 28.88 / 2 ) * 1 mm"
equation "d11 = ( 28.88 / 2 ) * 1 mm"
equation "d32 = ( 297 / 2 ) * 1 mm"
equation "d48 = 296 / 2"
equation "d59 = ( 297 / 2 ) * 1 mm"
